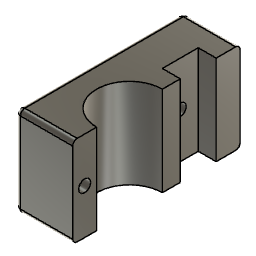
ConectorEstruturaGK_12 (Autodesk Fusion 360 design; units mm, degrees)
Autodesk Fusion 360 part; units mm, degrees
sketch "Esboço1" plane through (0, 0, 0) normal (0, 0, 1) x (1, 0, 0)
  line L0 (1.9999, 62) -> (2, 62)
  line L1 (15, 42) -> (21, 42)
  line L2 (15, 54) -> (15, 42)
  line L3 (2, 6) -> (2, 62)
  line L4 (1.9999, 62) -> (21, 62)
  line L5 (2, 6) -> (21, 6)
  line L6 (21, 62) -> (21, 54)
  line L7 (21, 54) -> (15, 54)
  line L8 (21, 14) -> (21, 6)
  line L9 (21, 42) -> (21, 36)
  arc A0 (21, 36) -> (21, 14) centre (21, 25) ccw
  dimension "d2" = 12
  dimension "d3" = 6
  dimension "d5" = 8
  dimension "d8" = 6
  dimension "d10" = 8
  dimension "d36" = 19
  dimension "d12" = 6
  dimension "d13" = 11
  constraint perpendicular L6 L7
  constraint perpendicular L2 L7
  constraint perpendicular L1 L2
  constraint vertical L8
  constraint perpendicular L5 L8
  constraint perpendicular L1 L9
  measures "d2" distance of L2.start L1.start
  measures "d3" distance of L6.end L2.start
  measures "d5" distance of L6.end L4.end
  measures "d8" distance of L1.start L1.end
  measures "d10" distance of L8.start L5.end
  measures "d36" distance of L4.end L0.end
  measures "d12" distance of L1.end L9.end
  measures "d13" distance of L9.end A0.centre
extrude "Extrusão1" add sketch "Esboço1" along normal blind 30
hole "Furo1" at (2, 48, 15) direction (1, 0, 0) diameter 4 depth 21 tip angle 180
hole "Furo2" at (2, 10, 15) direction (1, 0, 0) diameter 4 depth 21 tip angle 180
fillet "Arredondamento1" radius 1.5 8 edges at (11.5, 62, 30) (2, 62, 15) (2, 34, 30) (2, 6, 15) (11.5, 6, 30) (11.5, 6, 0) (2, 34, 0) (11.5, 62, 0)
